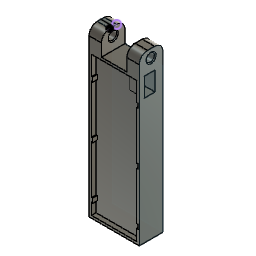
new cookie jar v7 (Autodesk Fusion 360 design; units mm, degrees)
Autodesk Fusion 360 part; units mm, degrees
sketch "Sketch1" plane through (0, 0, 0) normal (0, 0, 1) x (1, 0, 0)
  line L0 (0, 0) -> (60.75, 0)
  line L1 (60.75, 0) -> (60.75, 12.5)
  line L2 (60.75, 12.5) -> (0, 12.5)
  line L3 (0, 12.5) -> (0, 0)
  line L4 (0, 0) -> (3, 0)
  line L5 (3, 0) -> (3, 9.5)
  line L6 (60.75, 0) -> (57.75, 0)
  line L7 (57.75, 0) -> (57.75, 9.5)
  line L8 (57.75, 9.5) -> (3, 9.5)
  dimension "d1" = 60.75
  dimension "d2" = 12.5
  dimension "d3" = 3
  dimension "d4" = 9.5
  dimension "d5" = 3
  dimension "d6" = 9.5
  constraint coincident L0.start L3.end
  constraint horizontal L0
  constraint perpendicular L0 L1
  constraint perpendicular L1 L2
  constraint perpendicular L0 L3
  constraint perpendicular L3 L4
  constraint perpendicular L4 L5
  constraint perpendicular L1 L6
  constraint perpendicular L0 L7
  measures "d1" distance of L0.start L0.end
  measures "d2" distance of L0.end L1.end
  measures "d3" distance of L0.start L4.end
  measures "d4" distance of L4.end L5.end
  measures "d5" distance of L0.end L6.end
  measures "d6" distance of L6.end L7.end
extrude "Extrude1" add sketch "Sketch1" along normal blind 3
sketch "Sketch2" plane through (0, 0, 3) normal (0, 0, 1) x (-1, 0, 0)
  line L0 (-60.75, -12.5) -> (0, -12.5)
  line L1 (0, -12.5) -> (0, 0)
  line L2 (0, 0) -> (-60.75, 0)
  line L3 (-60.75, 0) -> (-60.75, -12.5)
  line L4 (0, 0) -> (-3, 0)
  line L5 (-3, 0) -> (-3, -9.5)
  line L6 (-60.75, 0) -> (-57.75, 0)
  line L7 (-57.75, 0) -> (-57.75, -9.5)
  line L8 (-57.75, -9.5) -> (-3, -9.5)
  dimension "d9" = 3
  dimension "d10" = 9.5
  dimension "d11" = 3
  dimension "d12" = 9.5
  constraint coincident L1.end L2.start
  constraint perpendicular L1 L4
  constraint perpendicular L4 L5
  constraint coincident L2.end L3.start
  constraint perpendicular L3 L6
  constraint perpendicular L6 L7
  measures "d9" distance of L1.end L4.end
  measures "d10" distance of L4.end L5.end
  measures "d11" distance of L2.end L6.end
  measures "d12" distance of L6.end L7.end
extrude "Extrude2" add sketch "Sketch2" along normal blind 171.5 contours L0 L1 L2 L3 L4 L5 L6 L7 L8
sketch "Sketch3" plane through (57.75, 0, 0) normal (-1, 0, 0) x (0, -1, 0)
  line L0 (-9.5, 3) -> (0, 3)
  line L1 (0, 3) -> (0, 174.5)
  line L2 (0, 174.5) -> (-9.5, 174.5)
  line L3 (-9.5, 174.5) -> (-9.5, 3)
  line L4 (-9.5, 174.5) -> (-9.5, 171.5)
  line L5 (-9.5, 171.5) -> (0, 171.5)
  line L6 (0, 171.5) -> (0, 174.5)
  line L7 (-9.5, 174.5) -> (0, 174.5)
  dimension "d15" = 3
  constraint coincident L2.end L3.start
  constraint perpendicular L2 L4
  constraint coincident L1 L5.end
  constraint perpendicular L1 L5
  constraint coincident L1.end L2.start
  measures "d15" distance of L2.end L4.end
extrude "Extrude3" add sketch "Sketch3" along normal blind 54.75 contours L1 L2 L3 L4 L5 L6 L7
sketch "Sketch4" plane through (0, 0, 0) normal (0, -1, 0) x (1, 0, 0)
  line L0 (57.75, 171.5) -> (57.75, 3)
  line L1 (57.75, 3) -> (3, 3)
  line L2 (3, 3) -> (3, 171.5)
  line L3 (3, 171.5) -> (57.75, 171.5)
  line L4 (60.75, 174.5) -> (0, 174.5)
  line L5 (0, 174.5) -> (0, 0)
  line L6 (0, 0) -> (60.75, 0)
  line L7 (60.75, 0) -> (60.75, 174.5)
  line L8 (57.75, 3) -> (57.75, 16.7)
  line L9 (57.75, 16.7) -> (57.75, 21.5)
  line L10 (57.75, 21.5) -> (57.75, 19.1)
  line L11 (59.25, 19.1) -> (59.25, 21.85)
  line L12 (59.25, 19.1) -> (59.25, 16.35)
  line L13 (59.25, 16.35) -> (57.75, 16.7)
  line L14 (59.25, 21.85) -> (57.75, 21.5)
  line L15 (59.25, 85.2) -> (57.75, 84.85)
  line L16 (59.25, 82.45) -> (59.25, 85.2)
  line L17 (59.25, 82.45) -> (59.25, 79.7)
  line L18 (59.25, 79.7) -> (57.75, 80.05)
  line L19 (57.75, 80.05) -> (57.75, 84.85)
  line L20 (59.25, 148.55) -> (57.75, 148.2)
  line L21 (59.25, 145.8) -> (59.25, 148.55)
  line L22 (59.25, 145.8) -> (59.25, 143.05)
  line L23 (59.25, 143.05) -> (57.75, 143.4)
  line L24 (57.75, 143.4) -> (57.75, 148.2)
  line L25 (4.5, 16.35) -> (3, 16.7)
  line L26 (4.5, 19.1) -> (4.5, 16.35)
  line L27 (4.5, 19.1) -> (4.5, 21.85)
  line L28 (4.5, 21.85) -> (3, 21.5)
  line L29 (3, 21.5) -> (3, 19.1)
  line L30 (3, 16.7) -> (3, 21.5)
  line L31 (3, 80.05) -> (3, 84.85)
  line L32 (4.5, 82.45) -> (4.5, 85.2)
  line L33 (4.5, 82.45) -> (4.5, 79.7)
  line L34 (4.5, 79.7) -> (3, 80.05)
  line L35 (4.5, 85.2) -> (3, 84.85)
  line L36 (4.5, 148.55) -> (3, 148.2)
  line L37 (3, 143.4) -> (3, 148.2)
  line L38 (4.5, 145.8) -> (4.5, 148.55)
  line L39 (4.5, 145.8) -> (4.5, 143.05)
  line L40 (4.5, 143.05) -> (3, 143.4)
  dimension "d18" = 13.7
  dimension "d19" = 4.8
  dimension "d21" = 1.5
  dimension "d24" = 4.8
  dimension "d25" = 4.8
  dimension "d26" = 4.8
  dimension "d27" = 1.5
  dimension "d28" = 4.8
  dimension "d29" = 4.8
  constraint coincident L0.end L1.start
  constraint perpendicular L1 L8
  constraint parallel L0 L9
  constraint parallel L0 L10
  measures "d18" distance of L0.end L8.end
  measures "d19" distance of L8.end L9.end
  measures "d21" distance of L10.end L11.start
  measures "d24" distance of L15.end L18.end
  measures "d25" distance of L20.end L23.end
  measures "d26" distance of L28.end L25.end
  measures "d27" distance of L29.end L26.start
  measures "d28" distance of L31.end L31.start
  measures "d29" distance of L37.start L36.end
extrude "Extrude4" cut sketch "Sketch4" against normal blind 9.5 contours L0 L20 L21 L22 L23 L24 | L2 L36 L37 L38 L39 L40 | L0 L15 L16 L17 L18 L19 | L2 L31 L32 L33 L34 L35 | L0 L9 L10 L11 L12 L13 L14 | L2 L25 L26 L27 L28 L29 L30
sketch "Sketch6" plane through (0, 9.5, 0) normal (0, -1, 0) x (1, 0, 0)
  line L0 (3, 171.5) -> (3, 3)
  line L1 (3, 3) -> (57.75, 3)
  line L2 (57.75, 3) -> (57.75, 16.7)
  line L3 (57.75, 16.7) -> (59.25, 16.35)
  line L4 (59.25, 16.35) -> (59.25, 21.85)
  line L5 (59.25, 21.85) -> (57.75, 21.5)
  line L6 (57.75, 21.5) -> (57.75, 80.05)
  line L7 (57.75, 80.05) -> (59.25, 79.7)
  line L8 (59.25, 79.7) -> (59.25, 85.2)
  line L9 (59.25, 85.2) -> (57.75, 84.85)
  line L10 (57.75, 84.85) -> (57.75, 143.4)
  line L11 (57.75, 143.4) -> (59.25, 143.05)
  line L12 (59.25, 143.05) -> (59.25, 148.55)
  line L13 (59.25, 148.55) -> (57.75, 148.2)
  line L14 (57.75, 148.2) -> (57.75, 171.5)
  line L15 (57.75, 171.5) -> (3, 171.5)
  line L16 (3, 3) -> (3, 16.7)
  line L17 (3, 16.7) -> (3, 21.5)
  line L18 (3, 16.7) -> (3, 19.1)
  line L19 (4.5, 19.1) -> (4.5, 16.35)
  line L20 (4.5, 16.35) -> (3, 16.7)
  line L21 (4.5, 19.1) -> (4.5, 21.85)
  line L22 (3, 21.5) -> (4.5, 21.85)
  line L23 (3, 80.05) -> (3, 82.45)
  line L24 (4.5, 82.45) -> (4.5, 79.7)
  line L25 (4.5, 79.7) -> (3, 80.05)
  line L26 (4.5, 82.45) -> (4.5, 85.2)
  line L27 (3, 84.85) -> (4.5, 85.2)
  line L28 (3, 80.05) -> (3, 84.85)
  line L29 (4.5, 145.8) -> (4.5, 143.05)
  line L30 (4.5, 145.8) -> (4.5, 148.55)
  line L31 (3, 148.2) -> (4.5, 148.55)
  line L32 (3, 143.4) -> (3, 148.2)
  line L33 (4.5, 143.05) -> (3, 143.4)
  dimension "d32" = 13.7
  dimension "d33" = 4.8
  dimension "d34" = 2.4
  dimension "d35" = 1.5
  dimension "d36" = 2.75
  dimension "d37" = 2.75
  dimension "d38" = 4.8
  dimension "d39" = 2.4
  dimension "d40" = 1.5
  dimension "d41" = 2.75
  dimension "d42" = 2.75
  dimension "d43" = 4.8
  dimension "d44" = 2.75
  dimension "d45" = 2.75
  constraint coincident L0.end L1.start
  constraint perpendicular L1 L16
  constraint parallel L0 L17
  constraint parallel L17 L18
  constraint parallel L23 L28
  measures "d32" distance of L0.end L16.end
  measures "d33" distance of L16.end L17.end
  measures "d34" distance of L16.end L18.end
  measures "d35" distance of L18.end L19.start
  measures "d36" distance of L19.start L19.end
  measures "d37" distance of L19.start L21.end
  measures "d38" distance of L27.start L23.start
  measures "d39" distance of L23.end L23.start
  measures "d40" distance of L24.start L23.end
  measures "d41" distance of L24.start L24.end
  measures "d42" distance of L24.start L26.end
  measures "d43" distance of L31.start L32.start
  measures "d44" distance of L29.start L29.end
  measures "d45" distance of L29.start L30.end
extrude "Extrude5" add sketch "Sketch6" along normal blind 9.5 contours L0 L29 L30 L31 L32 L33 | L0 L23 L24 L25 L26 L27 L28 | L0 L17 L18 L19 L20 L21 L22
extrude "Extrude6" cut 1 faces at (1, 0, 86.45) along direction (0, 1, 0) blind 4
move_body "Move1" bodies 1 to x (1, 0, 0) y (0, 1, 0) z (0, 0, 1) at (0, -4, 0)
extrude "Extrude7" add 1 faces at (40.5, 8.5, 58.1667) along direction (0, 1, 0) blind 20
sketch "Sketch7" plane through (60.75, 0, 0) normal (1, 0, 0) x (0, 1, 0)
  line L0 (0, 174.5) -> (0, 0)
  line L1 (0, 0) -> (28.5, 0)
  line L2 (28.5, 0) -> (28.5, 174.5)
  line L3 (28.5, 174.5) -> (0, 174.5)
  line L4 (0, 174.5) -> (6, 174.5)
  line L5 (6, 174.5) -> (19, 174.5)
  line L6 (19, 174.5) -> (19, 151.5)
  line L7 (19, 151.5) -> (6, 151.5)
  line L8 (6, 151.5) -> (6, 174.5)
  dimension "d52" = 6
  dimension "d53" = 13
  dimension "d54" = 23
  dimension "d55" = 13
  constraint coincident L0.start L3.end
  constraint perpendicular L0 L4
  constraint parallel L3 L5
  constraint perpendicular L5 L6
  constraint perpendicular L6 L7
  measures "d52" distance of L0.start L4.end
  measures "d53" distance of L4.end L5.end
  measures "d54" distance of L5.end L6.end
  measures "d55" distance of L6.end L7.end
extrude "Extrude8" cut sketch "Sketch7" against normal blind 18 contours L3 L5 L6 L7 L8
sketch "Sketch8" plane through (0, 0, 0) normal (0, -1, 0) x (1, 0, 0)
  line L0 (59.25, 79.7) -> (57.75, 80.05)
  line L1 (57.75, 80.05) -> (57.75, 21.5)
  line L2 (57.75, 21.5) -> (59.25, 21.85)
  line L3 (59.25, 21.85) -> (59.25, 16.35)
  line L4 (59.25, 16.35) -> (57.75, 16.7)
  line L5 (57.75, 16.7) -> (57.75, 3)
  line L6 (57.75, 3) -> (3, 3)
  line L7 (3, 3) -> (3, 16.7)
  line L8 (3, 16.7) -> (4.5, 16.35)
  line L9 (4.5, 16.35) -> (4.5, 21.85)
  line L10 (4.5, 21.85) -> (3, 21.5)
  line L11 (3, 21.5) -> (3, 80.05)
  line L12 (3, 80.05) -> (4.5, 79.7)
  line L13 (4.5, 79.7) -> (4.5, 85.2)
  line L14 (4.5, 85.2) -> (3, 84.85)
  line L15 (3, 84.85) -> (3, 143.4)
  line L16 (3, 143.4) -> (4.5, 143.05)
  line L17 (4.5, 143.05) -> (4.5, 148.55)
  line L18 (4.5, 148.55) -> (3, 148.2)
  line L19 (3, 148.2) -> (3, 171.5)
  line L20 (3, 171.5) -> (57.75, 171.5)
  line L21 (57.75, 171.5) -> (57.75, 148.2)
  line L22 (57.75, 148.2) -> (59.25, 148.55)
  line L23 (59.25, 148.55) -> (59.25, 143.05)
  line L24 (59.25, 143.05) -> (57.75, 143.4)
  line L25 (57.75, 143.4) -> (57.75, 84.85)
  line L26 (57.75, 84.85) -> (59.25, 85.2)
  line L27 (59.25, 85.2) -> (59.25, 79.7)
  line L28 (60.75, 174.5) -> (0, 174.5)
  line L29 (0, 174.5) -> (0, 0)
  line L30 (0, 0) -> (60.75, 0)
  line L31 (60.75, 0) -> (60.75, 174.5)
  line L32 (0, 3) -> (0, 50)
  line L33 (0, 3) -> (0, 26.5)
  line L34 (0, 26.5) -> (0, 28.9)
  line L35 (0, 26.5) -> (0, 24.1)
  line L36 (-1.5, 26.5) -> (-1.5, 29.25)
  line L37 (-1.5, 26.5) -> (-1.5, 23.75)
  line L38 (-1.5, 23.75) -> (0, 24.1)
  line L39 (-1.5, 29.25) -> (0, 28.9)
  dimension "d58" = 47
  dimension "d59" = 23.5
  dimension "d62" = 1.5
  constraint coincident L29 L32.start
  constraint parallel L29 L34
  constraint parallel L32 L35
  measures "d58" distance of L32.start L32.end
  measures "d59" distance of L32.start L33.end
  measures "d62" distance of L33.end L36.start
sketch "Sketch9" plane through (0, 28.5, 0) normal (0, 1, 0) x (-1, 0, 0)
  line L0 (-60.75, 0) -> (0, 0)
  line L1 (0, 0) -> (0, 174.5)
  line L2 (0, 174.5) -> (-60.75, 174.5)
  line L3 (-60.75, 174.5) -> (-60.75, 0)
sketch "Sketch10" plane through (0, 0, 0) normal (0, 0, -1) x (1, 0, 0)
  line L0 (60.75, 0) -> (0, 0)
  line L1 (0, 0) -> (0, -28.5)
  line L2 (0, -28.5) -> (60.75, -28.5)
  line L3 (60.75, -28.5) -> (60.75, 0)
  line L4 (0, -28.5) -> (30.375, -28.5)
  line L5 (30.375, -30) -> (28.375, -30)
  line L6 (30.375, -28.5) -> (28.875, -28.5)
  line L7 (28.875, -28.5) -> (28.375, -30)
  line L8 (30.375, -30) -> (32.375, -30)
  line L9 (30.375, -28.5) -> (31.875, -28.5)
  line L10 (32.375, -30) -> (31.875, -28.5)
  dimension "d65" = 30.375
  dimension "d66" = 1.5
  dimension "d67" = 2
  dimension "d68" = 1.5
  dimension "d69" = 2
  dimension "d70" = 1.5
  constraint coincident L1.end L2.start
  constraint perpendicular L1 L4
  measures "d65" distance of L1.end L4.end
  measures "d66" distance of L4.end L5.start
  measures "d67" distance of L5.start L5.end
  measures "d68" distance of L4.end L6.end
  measures "d69" distance of L5.start L8.end
  measures "d70" distance of L4.end L9.end
sketch "Sketch11" plane through (0, 0, 0) normal (0, 0, -1) x (1, 0, 0)
  line L0 (60.75, 0) -> (0, 0)
  line L1 (0, 0) -> (0, -28.5)
  line L2 (0, -28.5) -> (60.75, -28.5)
  line L3 (60.75, -28.5) -> (60.75, 0)
  line L4 (0, -28.5) -> (30.375, -28.5)
  line L5 (30.375, -33.5) -> (20.375, -33.5)
  line L6 (30.375, -28.5) -> (22.875, -28.5)
  line L7 (22.875, -28.5) -> (20.375, -33.5)
  line L8 (30.375, -33.5) -> (40.375, -33.5)
  line L9 (30.375, -28.5) -> (37.875, -28.5)
  line L10 (37.875, -28.5) -> (40.375, -33.5)
  dimension "d73" = 5
  dimension "d74" = 10
  dimension "d75" = 7.5
  dimension "d76" = 10
  dimension "d77" = 7.5
  constraint coincident L1.end L2.start
  constraint midpoint L2 L4.end
  measures "d73" distance of L4.end L5.start
  measures "d74" distance of L5.start L5.end
  measures "d75" distance of L4.end L6.end
  measures "d76" distance of L5.start L8.end
  measures "d77" distance of L4.end L9.end
extrude "Extrude10" add sketch "Sketch11" against normal blind 174.5 contours L2 L4 L5 L6 L7 L8 L9 L10
sketch "Sketch12" plane through (0, 0, 174.5) normal (0, 0, 1) x (-1, 0, 0)
  line L0 (-60.75, -6) -> (-42.75, -6)
  line L1 (-42.75, -6) -> (-42.75, -19)
  line L2 (-42.75, -19) -> (-60.75, -19)
  line L3 (-60.75, -19) -> (-60.75, -28.5)
  line L4 (-60.75, -28.5) -> (-37.875, -28.5)
  line L5 (-37.875, -28.5) -> (-40.375, -33.5)
  line L6 (-40.375, -33.5) -> (-20.375, -33.5)
  line L7 (-20.375, -33.5) -> (-22.875, -28.5)
  line L8 (-22.875, -28.5) -> (0, -28.5)
  line L9 (0, -28.5) -> (0, 0)
  line L10 (0, 0) -> (-60.75, 0)
  line L11 (-60.75, 0) -> (-60.75, -6)
  line L12 (-60.75, 0) -> (-45.75, 0)
  line L13 (-45.75, 0) -> (-45.75, -28.5)
  line L14 (-45.75, -28.5) -> (-60.75, -28.5)
  line L15 (-60.75, -28.5) -> (-60.75, 0)
  line L16 (0, 0) -> (-15, 0)
  line L17 (-15, 0) -> (-15, -28.5)
  line L18 (-15, -28.5) -> (0, -28.5)
  line L19 (0, -28.5) -> (0, 0)
  dimension "d80" = 15
  dimension "d81" = 15
  constraint horizontal L12
  constraint vertical L13
  constraint horizontal L14
  constraint vertical L15
  constraint coincident L4 L13.end
  constraint coincident L10.end L11.start
  constraint horizontal L16
  constraint vertical L17
  constraint horizontal L18
  constraint vertical L19
  constraint coincident L9.end L10.start
  measures "d80" distance of L10.end L12.end
  measures "d81" distance of L9.end L16.end
extrude "Extrude11" add sketch "Sketch12" along normal blind 25 contours L0 L10 L11 L12 L13 L15 | L2 L3 L4 L13 L14 L15 | L8 L9 L10 L16 L17 L18 L19
sketch "Sketch13" plane through (0, 19, 0) normal (0, -1, 0) x (1, 0, 0)
  line L0 (60.75, 151.5) -> (60.75, 199.5)
  line L1 (60.75, 199.5) -> (45.75, 199.5)
  line L2 (45.75, 199.5) -> (45.75, 174.5)
  line L3 (45.75, 174.5) -> (42.75, 174.5)
  line L4 (42.75, 174.5) -> (42.75, 151.5)
  line L5 (42.75, 151.5) -> (60.75, 151.5)
  line L6 (45.75, 174.5) -> (60.75, 174.5)
  constraint coincident L2.end L3.start
  constraint coincident L0 L6.end
  constraint perpendicular L0 L6
extrude "Extrude12" add sketch "Sketch13" along normal blind 13 contours L0 L1 L2 L6
fillet "Fillet1" radius 10 4 edges at (53.25, 28.5, 199.5) (7.5, 28.5, 199.5) (7.5, 0, 199.5) (53.25, 0, 199.5)
sketch "Sketch14" plane through (0, 0, 199.5) normal (0, 0, 1) x (-1, 0, 0)
  line L0 (0, -10) -> (-15, -10)
  line L1 (-15, -10) -> (-15, -18.5)
  line L2 (-15, -18.5) -> (0, -18.5)
  line L3 (0, -18.5) -> (0, -10)
  line L4 (-15, -10) -> (-15, -18.5)
  line L5 (-15, -10) -> (-15, -14.25)
  line L6 (-15, -14.25) -> (0, -14.25)
  dimension "d88" = 4.25
  constraint coincident L0.end L1.start
  constraint perpendicular L2 L5
  constraint midpoint L3 L6.end
  measures "d88" distance of L0.end L5.end
sketch "Sketch15" plane through (0, 0, 0) normal (-1, 0, 0) x (0, -1, 0)
  arc A0 (0, 189.5) -> (-10, 199.5) centre (-10, 189.5) ccw
  line L0 (-10, 199.5) -> (-18.5, 199.5)
  arc A1 (-18.5, 199.5) -> (-28.5, 189.5) centre (-18.5, 189.5) ccw
  line L1 (-28.5, 189.5) -> (-28.5, 0)
  line L2 (-28.5, 0) -> (0, 0)
  line L3 (0, 0) -> (0, 189.5)
  circle A2 centre (-14.25, 189.5) radius 5
extrude "Extrude13" cut sketch "Sketch15" against normal blind 60.75 contours A2
fillet "Fillet2" radius 1 4 edges at (60.75, 18.9116, 187.6919) (15, 18.9116, 187.6919) (45.75, 18.9116, 191.3081) (0, 18.9116, 191.3081)
sketch "Sketch16" plane through (60.75, 0, 0) normal (1, 0, 0) x (0, 1, 0)
  line L0 (19, 174.5) -> (19, 151.5)
  line L1 (19, 151.5) -> (6, 151.5)
  line L2 (6, 151.5) -> (6, 174.5)
  line L3 (6, 174.5) -> (19, 174.5)
  arc A0 (10, 199.5) -> (0, 189.5) centre (10, 189.5) ccw
  line L4 (0, 189.5) -> (0, 0)
  line L5 (0, 0) -> (28.5, 0)
  line L6 (28.5, 0) -> (28.5, 189.5)
  arc A1 (28.5, 189.5) -> (18.5, 199.5) centre (18.5, 189.5) ccw
  line L7 (18.5, 199.5) -> (10, 199.5)
  circle A2 centre (14.25, 189.5) radius 6
extrude "Extrude9" add sketch "Sketch10" against normal blind 174.5 contours L2 L4 L5 L6 L7 L8 L9 L10
